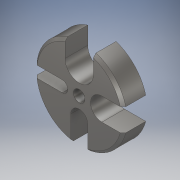
# Autodesk Inventor part: Table
Saved by Autodesk Inventor 2018 (Build 220112000, 112)
## iProperties
Created: 2017-12-20
Part Number: Table
Material: Stainless Steel
Document SubType Name: Modeling
Designer: 232963
Density: 8 g/cm^3
Appearance: Semi-Polished
Mass: 122.564 g
Surface Area: 62.2187 cm^2
Volume: 15.3205 cm^3
Author: 232963
Autodesk Inventor part; units mm, degrees
ref_plane "YZ Plane" through (0, 0, 0) normal (1, 0, 0) x (0, 1, 0)
ref_plane "XZ Plane" through (0, 0, 0) normal (0, 1, 0) x (-1, 0, 0)
ref_plane "XY Plane" through (0, 0, 0) normal (0, 0, 1) x (1, 0, 0)
sketch "Sketch1" plane through (0, 0, 0) normal (0, 0, 1) x (1, 0, 0)
  line L0 (4.7625, 0) -> (6.35, 0)
  line L1 (0, -3.175) -> (0, -3.2385)
  arc A0 (12.7, 6.35) -> (12.7, -6.35) centre (12.7, 0) ccw
  arc A1 (-7.9502, 14.2748) -> (7.9502, 14.2748) centre (0, 14.2748) ccw
  arc A2 (-9.525, -3.175) -> (-9.525, 3.175) centre (-9.525, 0) ccw
  arc A3 (4.7625, -11.0998) -> (-4.7625, -11.0998) centre (0, -11.0998) ccw
  circle A4 centre (0, 0) radius 3.2385
  line L2 (7.9502, 14.2748) -> (7.9502, 24.1237)
  line L3 (-7.9502, 14.2748) -> (-7.9502, 24.1237)
  line L4 (12.7, 6.35) -> (24.5934, 6.35)
  line L5 (12.7, -6.35) -> (24.5934, -6.35)
  arc A5 (24.5934, 6.35) -> (7.9502, 24.1237) centre (0, 0) ccw
  line L6 (-9.525, 3.175) -> (-25.2008, 3.175)
  line L7 (-9.525, -3.175) -> (-25.2008, -3.175)
  arc A6 (-7.9502, 24.1237) -> (-25.2008, 3.175) centre (0, 0) ccw
  line L8 (-4.7625, -11.0998) -> (-4.7625, -24.9495)
  line L9 (4.7625, -11.0998) -> (4.7625, -24.9495)
  arc A7 (-25.2008, -3.175) -> (-4.7625, -24.9495) centre (0, 0) ccw
  arc A8 (4.7625, -24.9495) -> (24.5934, -6.35) centre (0, 0) ccw
  dimension "d5" = 6.477
  dimension "d1" = 12.7
  dimension "d2" = 15.9004
  dimension "d3" = 6.35
  dimension "d4" = 9.525
  dimension "d6" = 11.0998
  dimension "d7" = 14.2748
  dimension "d8" = 12.7
  dimension "d9" = 9.525
  constraints: 20 end point, 17 point on circle, 8 centre point, 8 tangent, 4 point on line, 3 parallel, 2 coincident, 2 horizontal, 2 vertical, 1 perpendicular, 1 vertical alignment, 2 other
  measures "d1" diameter of A0
  measures "d2" diameter of A1
  measures "d3" diameter of A2
  measures "d4" diameter of A3
  measures "d6" distance of point (0, 0) A3.centre
  measures "d7" distance of point (0, 0) A1.centre
  measures "d8" distance of point (0, 0) A0.centre
  measures "d9" distance of point (0, 0) A2.centre
extrude "Extrusion1" add sketch "Sketch1" along normal blind 12.7
chamfer "Chamfer2" distance 1.524 angle 45 4 edges at (-19.6076, 16.1462, 12.7) (18.5405, 17.3612, 12.7) (17.3761, -18.5265, 12.7) (-18.5198, -17.3833, 12.7)
body "Solid1"
